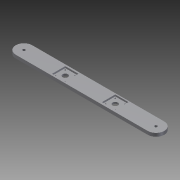
# Autodesk Inventor part: base side
Saved by Autodesk Inventor 2011 (Build 150239000, 239)
## iProperties
Created: 2010-04-19
Part Number: base side
Document SubType Name: Modeling
Designer: lucio
Density: 1 g/cm^3
Mass: 200.119 g
Surface Area: 553.994 cm^2
Volume: 200.119 cm^3
Author: lucio
Autodesk Inventor part; units mm, degrees
ref_plane "YZ Plane" through (0, 0, 0) normal (1, 0, 0) x (0, 1, 0)
ref_plane "XZ Plane" through (0, 0, 0) normal (0, 1, 0) x (-1, 0, 0)
ref_plane "XY Plane" through (0, 0, 0) normal (0, 0, 1) x (1, 0, 0)
sketch "Sketch1" plane through (0, 0, 0) normal (0, 0, 1) x (1, 0, 0)
  line L0 (0, 0) -> (400, 0)
  line L1 (400, 0) -> (400, 50)
  line L2 (400, 50) -> (0, 50)
  line L3 (0, 50) -> (0, 0)
  circle A0 centre (0, 25) radius 25
  circle A1 centre (400, 25) radius 25
  dimension "d0" = 400
  dimension "d1" = 50
  constraints: 8 end point, 2 midpoint, 2 parallel, 2 vertical alignment, 1 horizontal, 1 perpendicular, 4 other
  measures "d0" distance of L2.end L1.end
  measures "d1" distance of L1.end L0.end
extrude "Extrusion1" add sketch "Sketch1" along normal blind 10
sketch "Sketch2" plane through (0, 0, 10) normal (0, 0, 1) x (1, 0, 0)
  arc A0 (0, 50) -> (0, 0) centre (0, 25) ccw projected
  arc A1 (400, 0) -> (400, 50) centre (400, 25) ccw projected
  constraints: 2 coincident
hole "Hole1" at (0, 25, 10) at (400, 25, 10) direction (0, 0, -1) diameter 8 end through all
sketch "Sketch3" plane through (0, 0, 10) normal (0, 0, 1) x (1, 0, 0)
  circle A0 centre (0, 25) radius 4 projected
  circle A1 centre (400, 25) radius 4 projected
  point P0 (125, 25)
  point P1 (275, 26.5)
  dimension "d11" = 125
  dimension "d55" = 125
  measures "d11" distance of A0.centre point (125, 25)
  measures "d55" horizontal distance of A1.centre point (275, 26.5)
hole "Hole2" at (125, 25, 10) at (275, 26.5, 10) direction (0, 0, -1) diameter 16 end through all
sketch "Sketch4" plane through (0, 0, 10) normal (0, 0, 1) x (1, 0, 0)
  circle A0 centre (275, 26.5) radius 8 projected
  circle A1 centre (125, 25) radius 8 projected
  line L0 (110, 40) -> (140, 40)
  line L1 (140, 40) -> (140, 10)
  line L2 (140, 10) -> (110, 10)
  line L3 (110, 10) -> (110, 40)
  line L4 (260, 41.5) -> (290, 41.5)
  line L5 (290, 41.5) -> (290, 11.5)
  line L6 (290, 11.5) -> (260, 11.5)
  line L7 (260, 11.5) -> (260, 41.5)
  dimension "d22" = 30
  dimension "d23" = 30
  dimension "d26" = 30
  dimension "d27" = 30
  dimension "d30" = 15
  dimension "d32" = 15
  dimension "d34" = 15
  dimension "d36" = 15
  constraints: 16 end point, 4 parallel, 2 horizontal, 2 perpendicular
  measures "d22" distance of L1.end L2.end
  measures "d23" distance of L0.end L1.end
  measures "d26" distance of L5.end L6.end
  measures "d27" distance of L4.end L5.end
  measures "d30" distance from line of L0 A1.centre
  measures "d32" distance from line of A0.centre L4
  measures "d34" distance from line of L3 A1.centre
  measures "d36" distance from line of A0.centre L7
hole "Hole3" at (110, 10, 10) at (110, 40, 10) at (140, 40, 10) at (140, 10, 10) at (260, 11.5, 10) at (260, 41.5, 10) at (290, 41.5, 10) at (290, 11.5, 10) direction (0, 0, -1) diameter 4 end through all
sketch "Sketch5" plane through (0, 0, 10) normal (0, 0, 1) x (1, 0, 0)
  circle A0 centre (140, 10) radius 2 projected
  circle A1 centre (140, 40) radius 2 projected
  circle A2 centre (110, 40) radius 2 projected
  circle A3 centre (110, 10) radius 2 projected
  circle A4 centre (125, 25) radius 8 projected
  line L0 (105, 45) -> (145, 45)
  line L1 (145, 45) -> (145, 5)
  line L2 (145, 5) -> (105, 5)
  line L3 (105, 5) -> (105, 45)
  circle A5 centre (275, 26.5) radius 8 projected
  line L4 (255, 46.5) -> (295, 46.5)
  line L5 (295, 46.5) -> (295, 6.5)
  line L6 (295, 6.5) -> (255, 6.5)
  line L7 (255, 6.5) -> (255, 46.5)
  dimension "d45" = 40
  dimension "d46" = 40
  dimension "d47" = 20
  dimension "d48" = 20
  dimension "d51" = 40
  dimension "d52" = 40
  dimension "d53" = 20
  dimension "d54" = 20
  constraints: 16 end point, 4 parallel, 2 horizontal, 2 perpendicular
  measures "d45" distance of L1.end L2.end
  measures "d46" distance of L0.end L1.end
  measures "d47" distance from line of A4.centre L3
  measures "d48" distance from line of A4.centre L0
  measures "d51" distance of L5.end L6.end
  measures "d52" distance of L4.end L5.end
  measures "d53" distance from line of L7 A5.centre
  measures "d54" distance from line of L4 A5.centre
extrude "Extrusion2" cut sketch "Sketch5" against normal blind 5
equation "\"d55\" = d11"
equation "\"d32\" = d30"
equation "\"d36\" = d34"
body "Solid1"
